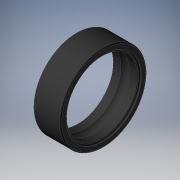
# Autodesk Inventor part: SKF_608-2RSL_PART2
Saved by Autodesk Inventor 2019 (Build 230136000, 136)
## iProperties
Created: 2022-07-08
Part Number: SKF_608-2RSL_PART2
Material: Generic
Catalog Web Link: www.cadenas.de
Description: -Deep groove ball bearings
Vendor: SKF
Document SubType Name: Modeling
Designer: psAdmin
Manufacturer: SKF
Mass: 12 g
Surface Area: 11.1165 cm^2
Volume: 0.819014 cm^3
Density: 1 g/cm^3
Appearance: PSOLRGB-175-175-175
Category: PARTsolutions
Company: SKF
Title: SKF_608-2RSL_PART2
Author: Cadenas PARTsolutions
Comments: Deep groove ball bearings
PSOL_IDENT_0: {$CADENAS_DATA/23d-libs/skf/bearings_units_and_housings/ball_bearings/deep_groove_ball_bearings/bb1_
PSOL_IDENT_1: 001_101.prj},202 {VTYP=3D},{NB=SKF_608-2RSL_PART2},{LINA=SKF_608-2RSL_PART2},{NN=BB1_001_101_PART2},
PSOL_IDENT_2: {NOPRJ=TRUE},{DATE=08.07.2022 10:24:27},{GEOMDATE=04.07.2022 10:54:51},{VERSION=},{LINEID=7700},{WBV
PSOL_IDENT_3: AR=},{WBNUMERIC=}  {NB=SKF_608-2RSL_PART2},{LINA=SKF_608-2RSL_PART2},{KT=DUMMY},{DESIGNATION=608-2RS
PSOL_IDENT_4: L},{R12=0.30},{DD=8.000},{D=22.000},{B=7.000},{C=},{CX=},{CXX=},{CA=0.000},{XXVARIANT=},{XXDESIGN=Si
PSOL_IDENT_5: ngle row},{XXSEALING=Low-friction seal on both sides},{DESIGN=dgbb2rs},{DESIGNIR=dgbb2rs},{VARIANT=}
PSOL_IDENT_6: ,{DD1=12.15},{DD2=10.55},{DD2X=},{DD2A=10.55},{D1=17.60},{D1X=0.00},{D2=19.2},{D2A=19.20},{D3=},{D3X=
PSOL_IDENT_7: },{D3A=0.000},{D4=},{HH=0.000},{BB=0.000},{BBX=},{BBA=0.000},{FF=},{R0MAX=0.000},{R0=0.000},{PITCH=1
PSOL_IDENT_8: 4.70},{DW=3.969},{DDAMIN=10.000},{DDAMAX=10.500},{DDBMIN=0.000},{DDBMAX=0.000},{DBMIN=0.000},{DAMAX=
PSOL_IDENT_9: 20.000},{BBAMIN=0.000},{CAMAX=0.000},{RAMAX=0.300},{LOAD1=3.450},{LOAD2=1.370},{LOAD3=0.057},{SPEED1=
PSOL_IDENT_10: 75000},{SPEED2=38000},{KR=0.025},{F0=12.000},{Z=7},{II=1},{MASS=0.012},{BEARING=608-2RSL},{RING=},{H
PSOL_IDENT_11: ELP=2.200},{HELP2=1.400},{DD1ALG=6.075},{YALG=6.075},{PITCH1=14.700},{DW1=3.969},{YALG1=8.800},{HALG
PSOL_IDENT_12: 1=2.200},{SH=5.275},{CU=0.606},{HALG=2.075},{B1=0},{SHIELDHELP=2},{D4A=0.000},{FFA=0.000},{RS1=},{HE
PSOL_IDENT_13: LP3=0}
NB: SKF_608-2RSL_PART2
NT: Deep groove ball bearings
NBSYN: SKF_$DESIGNATION._PART2
LINA: SKF_608-2RSL_PART2
CATALOG: SKF
DESIGNATION: 608-2RSL
R12: 0.3
DD: 8
D: 22
B: 7
XXDESIGN: Single row
XXSEALING: Low-friction seal on both sides
DD2: 10.55
D2: 19.2
LOAD1: 3.45
LOAD2: 1.37
LOAD3: 0.057
SPEED1: 75000
SPEED2: 38000
BEARING: 608-2RSL
SUPPLIER: SKF
ARTICLENO: SKF_608-2RSL_PART2
BOMINFO: SKF_608-2RSL_PART2
CREATOR: CADENAS GmbH
Autodesk Inventor part; units mm, degrees
ref_plane "YZ Plane" through (0, 0, 0) normal (1, 0, 0) x (0, 1, 0)
ref_plane "XZ Plane" through (0, 0, 0) normal (0, 1, 0) x (-1, 0, 0)
ref_plane "XY Plane" through (0, 0, 0) normal (0, 0, 1) x (1, 0, 0)
sketch "Sketch_9" plane through (0, 0, 0) normal (0, 0, 1) x (1, 0, 0)
  line L0 (50, 0) -> (-50, 0)
  line L1 (0, 10.7) -> (0, 9.6)
  line L2 (0, 9.6) -> (0.15, 9.6)
  arc A0 (0.45, 9.3) -> (0.15, 9.6) centre (0.15, 9.3) ccw
  line L3 (0.45, 9.3) -> (0.45, 9)
  line L4 (0.45, 9) -> (2.3974, 9)
  arc A1 (4.6026, 9) -> (2.3974, 9) centre (3.5, 7.35) ccw
  line L5 (4.6026, 9) -> (6.55, 9)
  line L6 (6.55, 9) -> (6.55, 9.3)
  arc A2 (6.85, 9.6) -> (6.55, 9.3) centre (6.85, 9.3) ccw
  line L7 (6.85, 9.6) -> (7, 9.6)
  line L8 (7, 9.6) -> (7, 10.7)
  arc A3 (7, 10.7) -> (6.7, 11) centre (6.7, 10.7) ccw
  line L9 (6.7, 11) -> (0.3, 11)
  arc A4 (0.3, 11) -> (0, 10.7) centre (0.3, 10.7) ccw
  constraints: 20 end point, 10 point on circle, 5 centre point
revolve "Revolution1" add sketch "Sketch_9" angle 360 about axis through (50, 0, 0) along (1, 0, 0)
body "Solid1"
